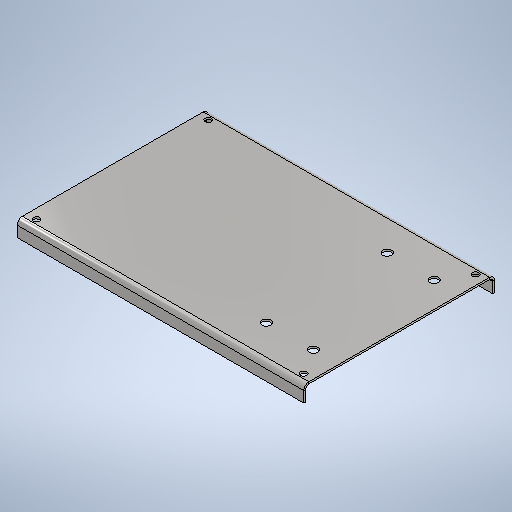
# Autodesk Inventor part: Purity pump plate
Saved by Autodesk Inventor 2025 (Build 290162010, 162A)
## iProperties
Created: 2024-12-06
Part Number: Purity pump plate
Material: Stainless Steel
Document SubType Name: Sheet Metal
Designer: pokla
Density: 8 g/cm^3
Sheet Metal Rule: AISI304 3mm Die 32
Appearance: Semi-Polished
Mass: 3632.62 g
Surface Area: 3083.54 cm^2
Volume: 454.078 cm^3
Flat Pattern Width: 33.7855 cm
Flat Pattern Length: 45 cm
Flat Pattern Area: 1520.35 cm^2
Sheet Metal Width: 337,855 mm
Sheet Metal Length: 450,000 mm
Sheet Metal Area: 152034,690 mm^2
Author: pokla
Autodesk Inventor part; units mm, degrees
ref_plane "YZ Plane" through (0, 0, 0) normal (1, 0, 0) x (0, 1, 0)
ref_plane "XZ Plane" through (0, 0, 0) normal (0, 1, 0) x (-1, 0, 0)
ref_plane "XY Plane" through (0, 0, 0) normal (0, 0, 1) x (1, 0, 0)
sketch "Sketch1" plane through (0, 0, 0) normal (0, 0, 1) x (1, 0, 0)
  line L0 (-225, 150) -> (225, 150)
  line L1 (225, 150) -> (225, -150)
  line L2 (225, -150) -> (-225, -150)
  line L3 (-225, -150) -> (-225, 150)
  line L4 (-225, 150) -> (225, -150) construction
  point P0 (0, 0)
  point P1 (0, 0)
  dimension "d0" = 450
  dimension "d1" = 300
  measures "d0" distance of L0.start L0.end
  measures "d1" distance of L2.end L0.start
extrude "Plate1" add sketch "Sketch1" against normal blind 3
sketch "Sketch2" plane through (0, 0, 0) normal (0, 0, 1) x (1, 0, 0)
  line L0 (111, 95) -> (185, 95) construction
  line L1 (185, 95) -> (185, -95) construction
  line L2 (185, -95) -> (111, -95) construction
  line L3 (111, -95) -> (111, 95) construction
  line L4 (225, -150) -> (225, 150) projected
  point P0 (0, 0)
  point P1 (111, 0)
  dimension "d3" = 74
  dimension "d4" = 190
  dimension "d5" = 40
  constraints: 8 end point, 4 coincident, 2 parallel, 1 horizontal, 1 horizontal alignment, 1 midpoint, 1 perpendicular
  measures "d3" distance of L0.start L0.end
  measures "d4" distance of L0.end L1.end
  measures "d5" distance between parallel lines of L4 L1
hole "Hole1" at (111, 95, 0) at (185, 95, 0) at (111, -95, 0) at (185, -95, 0) direction (0, 0, -1) diameter 14 end through all
sketch "Sketch3" plane through (0, 0, 0) normal (0, 0, 1) x (1, 0, 0)
  line L0 (-210, 135) -> (210, 135) construction
  line L1 (210, 135) -> (210, -135) construction
  line L2 (210, -135) -> (-210, -135) construction
  line L3 (-210, -135) -> (-210, 135) construction
  line L4 (-210, 135) -> (210, -135) construction
  point P0 (0, 0)
  point P1 (0, 0)
  dimension "d14" = 270
  dimension "d15" = 420
  constraints: 10 end point, 5 coincident, 2 parallel, 1 horizontal, 1 midpoint, 1 perpendicular
  measures "d14" distance of L2.end L0.start
  measures "d15" distance of L0.start L0.end
hole "Hole2" at (-210, 135, 0) at (210, 135, 0) at (210, -135, 0) at (-210, -135, 0) direction (0, 0, -1) diameter 10 end through all
sketch "Sketch4" plane through (-225, -147, 0) normal (0, -1, 0) x (1, 0, 0)
  line L0 (450, 0) -> (0, 0)
  line L1 (0, 0) -> (0, -25)
  line L2 (0, -25) -> (450, -25)
  line L3 (450, -25) -> (450, 0)
  constraints: 6 end point, 1 horizontal, 1 perpendicular, 1 vertical
edge flange "Flange1" height 25 angle 90 thickness 3 bend radius 5 thickness toward (0, -1, 0) relief round relief width 3 relief depth 1.5 corner gap 5 corner form 0 edges at (0, -150, -3) (0, 150, -3) wall of the first edge with corners at (225, -147, 0) (-225, -147, 0) (-225, -147, -25) (225, -147, -25)
bend "Bend1"
corner "Corner1"
equation "\"d11\" = Thickness"
equation "\"d2\" = Thickness"
equation "\"d23\" = BendReliefWidth"
equation "\"d24\" = BendReliefDepth"
equation "\"d25\" = MinimumRemnant"
equation "\"d26\" = TransitionRadius"
equation "\"d29\" = BendRadius"
equation "\"d30\" = CornerReliefSize"
equation "\"d31\" = GapSize"
equation "\"d32\" = JacobiRadiusSize"
equation "\"BendReliefWidth\" = Thickness"
equation "\"BendReliefDepth\" = 0.5 * Thickness"
equation "\"CornerReliefSize\" = 4 * Thickness"
equation "\"MinimumRemnant\" = 2 * Thickness"
equation "\"TransitionRadius\" = BendRadius"
equation "\"JacobiRadiusSize\" = BendRadius"
equation "\"GapSize\" = Thickness"
equation "\"Thickness\" = 3"
equation "\"BendRadius\" = 5"
body "Solid1"
